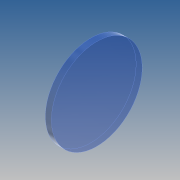
# Autodesk Inventor part: F117Lens30mm
Saved by Autodesk Inventor 2017 (Build 210142000, 142)
## iProperties
Created: 2018-01-17
Part Number: F117Lens30mm
Material: Glass
Document SubType Name: Modeling
Designer: serge.amoos
Density: 2.18 g/cm^3
Appearance: Clear - Blue
Author: serge.amoos
Autodesk Inventor part; units mm, degrees
ref_plane "YZ Plane" through (0, 0, 0) normal (1, 0, 0) x (0, 1, 0)
ref_plane "XZ Plane" through (0, 0, 0) normal (0, 1, 0) x (-1, 0, 0)
ref_plane "XY Plane" through (0, 0, 0) normal (0, 0, 1) x (1, 0, 0)
sketch "Sketch1" plane through (0, 0, 0) normal (0, 0, 1) x (1, 0, 0)
  line L0 (-14.4949, 0) -> (51.1241, 0) construction
  line L1 (0, -3.0207) -> (0, 18.1241) construction
  arc A0 (-2, 15) -> (-4.5, 0) centre (41.75, 0) ccw
  line L2 (-2, 15) -> (0, 15)
  line L3 (0, 15) -> (0, 0)
  line L4 (-4.5, 0) -> (0, 0)
  dimension "d0" = 30
  dimension "d1" = 2
  dimension "d2" = 4.5
  constraints: 6 end point, 2 collinear, 2 point on circle, 2 point on line, 1 centre point, 1 horizontal
  measures "d0" diameter of L2 L0
  measures "d1" distance of L2.start L2.end
  measures "d2" distance from line of L1 L4.start
revolve "Revolution1" add sketch "Sketch1" angle 360 about axis through (-10, 0, 0) along (1, 0, 0)
body "Solid1"
